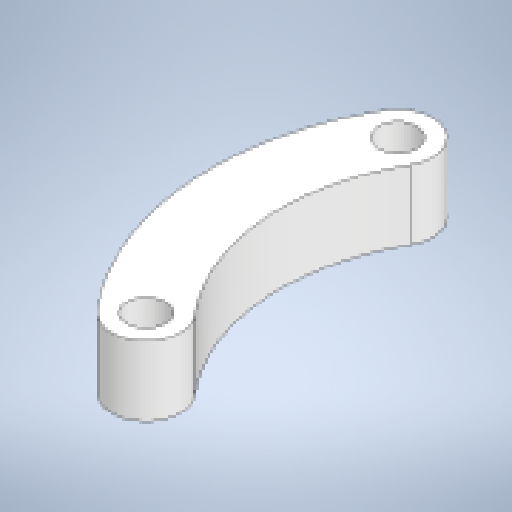
# Autodesk Inventor part: Top Plate
Saved by Autodesk Inventor 2023.2 (Build 272271000, 271)
## iProperties
Created: 2022-12-28
Part Number: Top Plate
Material: Nylon 6/6
Document SubType Name: Modeling
Designer: Nathan Cai
Mass: 37.6209 g
Surface Area: 285.387 cm^2
Volume: 40.0223 cm^3
Density: 1.13 g/cm^3
Appearance: Smooth - White
Author: Nathan Cai
Autodesk Inventor part; units mm, degrees
ref_plane "YZ Plane" through (0, 0, 0) normal (1, 0, 0) x (0, 1, 0)
ref_plane "XZ Plane" through (0, 0, 0) normal (0, 1, 0) x (-1, 0, 0)
ref_plane "XY Plane" through (0, 0, 0) normal (0, 0, 1) x (1, 0, 0)
sketch "Sketch1" plane through (0, 0, 0) normal (0, 1, 0) x (-1, 0, 0)
  circle A0 centre (0, 0) radius 73.025
  line L0 (0, 0) -> (0, -73.025) construction
  line L1 (0, 0) -> (-12.6807, -71.9156)
  line L2 (0, 0) -> (12.6807, -71.9156)
  line L3 (0, 0) -> (72.3143, -10.1631)
  line L4 (0, 0) -> (64.4772, -34.2832)
  line L5 (0, 0) -> (32.0121, 65.6344)
  line L6 (0, 0) -> (52.5298, 50.7274)
  line L7 (0, 0) -> (-52.5298, 50.7274)
  line L8 (0, 0) -> (-32.0121, 65.6344)
  line L9 (0, 0) -> (-64.4772, -34.2832)
  line L10 (0, 0) -> (-72.3143, -10.1631)
  circle A1 centre (0, 0) radius 69.85
  arc A2 (4.7597, -69.6876) -> (-4.7597, -69.6876) centre (0, -69.85) ccw
  arc A3 (67.7477, -17.0079) -> (64.806, -26.0614) centre (66.4313, -21.5848) ccw
  arc A4 (37.1107, 59.1762) -> (44.8121, 53.5808) centre (41.0568, 56.5098) ccw
  arc A5 (-44.8121, 53.5808) -> (-37.1107, 59.1762) centre (-41.0568, 56.5098) ccw
  arc A6 (-64.806, -26.0614) -> (-67.7477, -17.0079) centre (-66.4313, -21.5848) ccw
  point P0 (61.6739, -32.7926)
  point P1 (69.1702, -9.7212)
  point P2 (50.2459, 48.5219)
  point P3 (30.6202, 62.7808)
  point P4 (-30.6202, 62.7808)
  point P5 (-50.2459, 48.5219)
  point P6 (-69.1702, -9.7212)
  point P7 (-61.6739, -32.7926)
  point P8 (-12.1293, -68.7888)
  point P9 (12.1293, -68.7888)
  point P10 (64.806, -26.0614)
  point P11 (67.7477, -17.0079)
  point P12 (44.8121, 53.5808)
  point P13 (37.1107, 59.1762)
  point P14 (-37.1107, 59.1762)
  point P15 (-67.7477, -17.0079)
  dimension "d0" = 146.05
  dimension "d1" = 10
  dimension "d4" = 360
  dimension "d6" = 3.175
  dimension "d10" = 9.525
  dimension "d13" = 360
  constraints: 22 end point, 15 point on circle, 7 centre point, 4 coincident, 1 point on line, 1 symmetric about line, 1 vertical, 45 other
  measures "d0" diameter of A0
  measures "d1" angle of L0 L1
  measures "d6" radial gap between concentric circles of A0 A1
  measures "d10" diameter of A2
extrude "Extrusion1" add sketch "Sketch1" along normal blind 6.35 contours A0 L3 A1 L6 | L5 A1 L8 A0 | A1 L3 L6 | L6 L5 A1 A4 | A0 L2 A1 L4 | A1 A3 L4 L3 | L5 L8 A1 | L2 A1 A2 L1 | L4 A1 L2 | L10 A1 L7 | L7 A1 A5 L8 | L1 A1 L9 | L9 A1 A6 L10 | L7 A1 L10 A0 | L1 A0 L9 A1
fillet "Fillet1" radius 1.5875 30 edges at (30.6202, 3.175, 62.7808) (32.0121, 3.175, 65.6344) (-30.6202, 3.175, 62.7808) (-32.0121, 3.175, 65.6344) (-52.5298, 3.175, 50.7274) (-50.2459, 3.175, 48.5219) (52.5298, 3.175, 50.7274) (50.2459, 3.175, 48.5219) (64.4772, 3.175, -34.2832) (61.6739, 3.175, -32.7926) (72.3143, 3.175, -10.1631) (69.1702, 3.175, -9.7212) (12.6807, 3.175, -71.9156) (12.1293, 3.175, -68.7888) (-12.6807, 3.175, -71.9156) (-12.1293, 3.175, -68.7888) (-72.3143, 3.175, -10.1631) (-69.1702, 3.175, -9.7212) (-64.4772, 3.175, -34.2832) (-61.6739, 3.175, -32.7926) (37.1107, 3.175, 59.1762) (44.8121, 3.175, 53.5808) (-44.8121, 3.175, 53.5808) (-37.1107, 3.175, 59.1762) (-64.806, 3.175, -26.0614) (-67.7477, 3.175, -17.0079) (4.7597, 3.175, -69.6876) (-4.7597, 3.175, -69.6876) (67.7477, 3.175, -17.0079) (64.806, 3.175, -26.0614)
sketch "Sketch5" plane through (0, 6.35, 0) normal (0, 1, 0) x (1, 0, 0)
  line L0 (0, 0) -> (0, 65.0875) construction
  arc A0 (-4.554, 68.4564) -> (4.554, 68.4564) centre (0, 69.85) ccw projected
  circle A1 centre (0, 50.8) radius 22.225 construction
  arc A2 (63.6995, 35.7075) -> (14.2757, 71.616) centre (0, 0) ccw projected
  circle A3 centre (-24.6062, 60.325) radius 1.7526
  circle A4 centre (-24.6062, 60.325) radius 3.175
  circle A5 centre (-22.225, 34.925) radius 3.175
  circle A6 centre (-22.225, 34.925) radius 1.7526
  circle A7 centre (24.6062, 60.325) radius 1.7526
  circle A8 centre (24.6062, 60.325) radius 3.175
  circle A9 centre (22.225, 34.925) radius 3.175
  circle A10 centre (22.225, 34.925) radius 1.7526
  arc A11 (6.2133, 69.5731) -> (4.554, 68.4564) centre (6.0721, 67.9919) ccw projected
  arc A12 (6.2133, 69.5731) -> (4.554, 68.4564) centre (6.0721, 67.9919) ccw
  arc A13 (-4.554, 68.4564) -> (-6.2133, 69.5731) centre (-6.0721, 67.9919) ccw projected
  arc A14 (-4.554, 68.4564) -> (-6.2133, 69.5731) centre (-6.0721, 67.9919) ccw
  arc A15 (-12.4019, 70.3348) -> (-10.5977, 69.0414) centre (-10.8385, 70.6105) ccw projected
  arc A16 (10.5977, 69.0414) -> (12.4019, 70.3348) centre (10.8385, 70.6105) ccw projected
  arc A17 (10.5977, 69.0414) -> (6.2133, 69.5731) centre (0, 0) ccw projected
  arc A18 (10.5977, 69.0414) -> (11.9875, 69.515) centre (10.8385, 70.6105) ccw
  arc A19 (-6.2133, 69.5731) -> (-10.5977, 69.0414) centre (0, 0) ccw
  arc A20 (-14.2757, 71.616) -> (-63.6995, 35.7075) centre (0, 0) ccw projected
  line L1 (-28.4451, 67.2572) -> (-25.3861, 34.6286) construction
  line L2 (-22.7046, 31.7864) -> (-3.3572, 28.83) construction
  line L3 (28.4451, 67.2572) -> (25.3861, 34.6286) construction
  line L4 (22.7046, 31.7864) -> (3.3572, 28.83) construction
  circle A21 centre (0, 0) radius 73.025
  circle A22 centre (0, 50.8) radius 19.05 construction
  arc A23 (-27.365, 61.8966) -> (-24.6436, 32.868) centre (-5.295, 49.3238) ccw
  arc A24 (-21.8475, 58.7534) -> (-19.8064, 36.982) centre (-5.295, 49.3238) ccw
  point P0 (-63.6995, 35.7075)
  point P1 (-9.2869, 69.2299)
  point P2 (9.2869, 69.2299)
  point P3 (-5.0165, 69.1776)
  point P4 (5.0165, 69.1776)
  point P5 (14.2757, 71.616)
  dimension "d40" = 44.45
  dimension "d41" = 3.5052
  dimension "d42" = 6.35
  dimension "d43" = 9.525
  dimension "d44" = 24.6062
  dimension "d45" = 6.35
  dimension "d46" = 3.5052
  dimension "d47" = 15.875
  dimension "d48" = 22.225
  dimension "d70" = 38.1
  dimension "d72" = 25.4
  dimension "d73" = 19.05
  constraints: 30 point on circle, 16 centre point, 10 end point, 9 coincident, 9 symmetric about line, 9 tangent, 1 point on line, 1 vertical, 8 other
  measures "d40" diameter of A1
  measures "d41" diameter of A3
  measures "d42" diameter of A4
  measures "d43" vertical distance of A1.centre A3.centre
  measures "d44" horizontal distance of A1.centre A3.centre
  measures "d45" diameter of A5
  measures "d46" diameter of A6
  measures "d47" vertical distance of A1.centre A6.centre
  measures "d48" horizontal distance of A1.centre A6.centre
  measures "d70" diameter of A22
  measures "d72" radius of A23
  measures "d73" radius of A24
extrude "Extrusion3" cut sketch "Sketch5" against normal blind 25.4 contours A21 A20 A2 | A3 | A6 | A7 | A8 | A9 | A10
equation "\"d45\" = d42"
equation "\"d46\" = d41"
body "Solid1"
